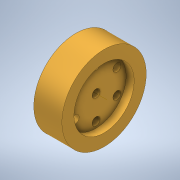
# Autodesk Inventor part: valve
Saved by Autodesk Inventor 2021.1 (Build 251245000, 245)
## iProperties
Created: 2020-08-29
Part Number: valve
Material: Brass, Soft Yellow
Document SubType Name: Sheet Metal
Designer: Vamshi
Density: 8.47 g/cm^3
Sheet Metal Rule: Default
Appearance: Brass - Satin
Mass: 2177.62 g
Surface Area: 367.667 cm^2
Volume: 257.099 cm^3
Author: Vamshi
Autodesk Inventor part; units mm, degrees
ref_plane "YZ Plane" through (0, 0, 0) normal (1, 0, 0) x (0, 1, 0)
ref_plane "XZ Plane" through (0, 0, 0) normal (0, 1, 0) x (-1, 0, 0)
ref_plane "XY Plane" through (0, 0, 0) normal (0, 0, 1) x (1, 0, 0)
sketch "Sketch1" plane through (0, 0, 0) normal (0, 0, 1) x (1, 0, 0)
  circle A0 centre (0, 0) radius 53.34
  dimension "d0" = 106.68
  constraints: 1 centre point, 1 coincident
  measures "d0" diameter of A0
extrude "Extrusion1" add sketch "Sketch1" along normal blind 35.56
sketch "Sketch2" plane through (0, 0, 35.56) normal (0, 0, 1) x (1, 0, 0)
  circle A0 centre (0, 0) radius 38.1
  dimension "d3" = 76.2
  constraints: 1 centre point, 1 coincident
  measures "d3" diameter of A0
extrude "Extrusion2" cut sketch "Sketch2" against normal blind 10.16
sketch "Sketch3" plane through (0, 0, 25.4) normal (0, 0, 1) x (1, 0, 0)
  line L0 (-74.676, 0) -> (74.676, 0) construction
  line L1 (0, -74.676) -> (0, 74.676) construction
  circle A0 centre (0, 0) radius 30.48
  circle A1 centre (0, 30.48) radius 5.08
  circle A2 centre (-26.3965, 15.24) radius 5.08
  circle A3 centre (-26.3965, -15.24) radius 5.08
  circle A4 centre (0, -30.48) radius 5.08
  circle A5 centre (26.3965, -15.24) radius 5.08
  circle A6 centre (26.3965, 15.24) radius 5.08
  circle A7 centre (0, 0) radius 5.08
  dimension "d6" = 60.96
  dimension "d7" = 10.16
  dimension "d10" = 360
  dimension "d14" = 10.16
  constraints: 7 centre point, 2 coincident, 1 point on line, 1 vertical alignment, 15 other
  measures "d7" diameter of A1
  measures "d14" diameter of A7
extrude "Extrusion3" cut sketch "Sketch3" against normal through all contours A6 A0 | A0 A6 | A5 A0 | A0 A5 | A1 A0 | A0 A1 | A4 A0 | A0 A4 | A2 A0 | A0 A2 | A3 A0 | A0 A3 | A7
sketch "Sketch4" plane through (0, 0, 0) normal (1, 0, 0) x (0, 1, 0)
  line L0 (-38.1, 25.4) -> (38.1, 25.4) projected
  line L1 (53.34, 35.56) -> (-53.34, 35.56) projected
  line L2 (53.34, 0) -> (-53.34, 0) projected
  line L3 (-5.08, 25.4) -> (-5.08, 0) projected
  line L4 (-5.08, 0) -> (-25.4, 0) projected
  line L5 (-25.4, 0) -> (-25.4, 25.4) projected
  line L6 (-25.4, 25.4) -> (-5.08, 25.4) projected
  line L7 (5.08, 0) -> (5.08, 25.4) projected
  line L8 (5.08, 25.4) -> (25.4, 25.4) projected
  line L9 (25.4, 25.4) -> (25.4, 0) projected
  line L10 (25.4, 0) -> (5.08, 0) projected
  line L11 (53.34, 35.56) -> (53.34, 0) projected
  line L12 (53.34, 0) -> (35.56, 0) projected
  line L13 (35.56, 0) -> (35.56, 25.4) projected
  line L14 (35.56, 25.4) -> (38.1, 25.4) projected
  line L15 (38.1, 25.4) -> (38.1, 35.56) projected
  line L16 (38.1, 35.56) -> (53.34, 35.56) projected
  line L17 (-53.34, 0) -> (-53.34, 35.56) projected
  line L18 (-53.34, 35.56) -> (-38.1, 35.56) projected
  line L19 (-38.1, 35.56) -> (-38.1, 25.4) projected
  line L20 (-38.1, 25.4) -> (-35.56, 25.4) projected
  line L21 (-35.56, 25.4) -> (-35.56, 0) projected
  line L22 (-35.56, 0) -> (-53.34, 0) projected
  line L23 (-5.08, 25.4) -> (-5.08, 0) projected
  line L24 (-5.08, 0) -> (-25.4, 0) projected
  line L25 (-25.4, 0) -> (-25.4, 25.4) projected
  line L26 (-25.4, 25.4) -> (-5.08, 25.4) projected
  line L27 (5.08, 0) -> (5.08, 25.4) projected
  line L28 (5.08, 25.4) -> (25.4, 25.4) projected
  line L29 (25.4, 25.4) -> (25.4, 0) projected
  line L30 (25.4, 0) -> (5.08, 0) projected
  line L31 (53.34, 35.56) -> (53.34, 0) projected
  line L32 (53.34, 0) -> (35.56, 0) projected
  line L33 (35.56, 0) -> (35.56, 25.4) projected
  line L34 (35.56, 25.4) -> (38.1, 25.4) projected
  line L35 (38.1, 25.4) -> (38.1, 35.56) projected
  line L36 (38.1, 35.56) -> (53.34, 35.56) projected
  line L37 (-53.34, 0) -> (-53.34, 35.56) projected
  line L38 (-53.34, 35.56) -> (-38.1, 35.56) projected
  line L39 (-38.1, 35.56) -> (-38.1, 25.4) projected
  line L40 (-38.1, 25.4) -> (-35.56, 25.4) projected
  line L41 (-35.56, 25.4) -> (-35.56, 0) projected
  line L42 (-35.56, 0) -> (-53.34, 0) projected
  line L43 (-5.08, 25.4) -> (-5.08, 0) projected
  line L44 (-5.08, 0) -> (-25.4, 0) projected
  line L45 (-25.4, 0) -> (-25.4, 25.4) projected
  line L46 (-25.4, 25.4) -> (-5.08, 25.4) projected
  line L47 (5.08, 0) -> (5.08, 25.4) projected
  line L48 (5.08, 25.4) -> (25.4, 25.4) projected
  line L49 (25.4, 25.4) -> (25.4, 0) projected
  line L50 (25.4, 0) -> (5.08, 0) projected
  line L51 (53.34, 35.56) -> (53.34, 0) projected
  line L52 (53.34, 0) -> (35.56, 0) projected
  line L53 (35.56, 0) -> (35.56, 25.4) projected
  line L54 (35.56, 25.4) -> (38.1, 25.4) projected
  line L55 (38.1, 25.4) -> (38.1, 35.56) projected
  line L56 (38.1, 35.56) -> (53.34, 35.56) projected
  line L57 (-53.34, 0) -> (-53.34, 35.56) projected
  line L58 (-53.34, 35.56) -> (-38.1, 35.56) projected
  line L59 (-38.1, 35.56) -> (-38.1, 25.4) projected
  line L60 (-38.1, 25.4) -> (-35.56, 25.4) projected
  line L61 (-35.56, 25.4) -> (-35.56, 0) projected
  line L62 (-35.56, 0) -> (-53.34, 0) projected
  line L63 (53.34, 35.56) -> (-53.34, 35.56) projected
  line L64 (53.34, 0) -> (-53.34, 0) projected
  line L65 (53.34, 0) -> (-53.34, 0) construction
  line L66 (12.7, 0) -> (12.7, 35.56) construction
  line L67 (-12.7, 0) -> (-12.7, 35.56) construction
  line L68 (0, -7.112) -> (0, 42.672) projected
  line L69 (48.26, 0) -> (12.7, 0)
  line L70 (12.7, 0) -> (12.7, 10.16)
  line L71 (12.7, 10.16) -> (48.26, 10.16)
  line L72 (48.26, 10.16) -> (48.26, 0)
  point P0 (0, 0)
  point P1 (0, 35.56)
  point P2 (0, 25.4)
  dimension "d15" = 25.4
  dimension "d16" = 10.16
  dimension "d17" = 5.08
  dimension "d18" = 7.62
  constraints: 12 end point, 3 parallel, 2 perpendicular, 2 point on line, 1 horizontal, 5 other
  measures "d15" distance between parallel lines of L66 L67
  measures "d16" distance of L69.end L70.end
  measures "d17" distance between parallel lines of L11 L72
  measures "d18" distance between parallel lines of L7 L70
revolve "Revolution1" cut sketch "Sketch4" angle 360 about axis through (0, 0, -10) along (0, 0, 1) contours L1 L15 L0 L68
equation "\"BendRadius\" = Thickness"
equation "\"BendReliefWidth\" = Thickness"
equation "\"BendReliefDepth\" = 0.5 * Thickness"
equation "\"CornerReliefSize\" = 4 * Thickness"
equation "\"MinimumRemnant\" = 2 * Thickness"
equation "\"TransitionRadius\" = BendRadius"
equation "\"JacobiRadiusSize\" = BendRadius"
equation "\"GapSize\" = Thickness"
equation "\"Thickness\" = 3.048"
body "Solid1"
